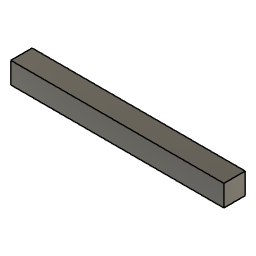
Tensile_ (2) (Autodesk Fusion 360 design; units mm, degrees)
Autodesk Fusion 360 part; units mm, degrees
sketch "Sketch1" plane through (0, 0, 0) normal (0, 1, 0) x (1, 0, 0)
  line L0 (-50, -50) -> (50, -50)
  line L1 (50, -50) -> (50, -40)
  line L2 (50, -40) -> (-50, -40)
  line L3 (-50, -40) -> (-50, -50)
  dimension "d1" = 100
  dimension "d2" = 10
  constraint horizontal L0
  constraint vertical L1
  constraint horizontal L2
  constraint vertical L3
  measures "d1" distance of L0.start L0.end
  measures "d2" distance of L0.end L1.end
extrude "Extrude1" add sketch "Sketch1" along normal blind 10
